Autodesk Fusion 360 part; units mm, degrees
(part 2 of 2)
  arc A402 (23.1836, 18.6599) -> (23.1836, 18.8885) centre (23.1836, 18.7742) ccw
  arc A403 (35.7225, 18.2179) -> (35.7225, 18.4465) centre (35.7225, 18.3322) ccw
  arc A404 (35.7225, 18.2179) -> (35.7225, 18.4465) centre (35.7225, 18.3322) ccw
  arc A405 (35.7225, 18.4465) -> (35.7225, 18.2179) centre (35.7225, 18.3322) ccw
  arc A406 (25.9333, 19.1335) -> (25.9333, 19.3621) centre (25.9333, 19.2478) ccw
  arc A407 (35.7225, 18.4465) -> (35.7225, 18.2179) centre (35.7225, 18.3322) ccw
  arc A408 (25.9333, 19.3621) -> (25.9333, 19.1335) centre (25.9333, 19.2478) ccw
  arc A409 (25.9333, 19.3621) -> (25.9333, 19.1335) centre (25.9333, 19.2478) ccw
  arc A410 (25.9333, 19.1335) -> (25.9333, 19.3621) centre (25.9333, 19.2478) ccw
  arc A411 (35.725, 17.5677) -> (35.725, 17.7963) centre (35.725, 17.682) ccw
  arc A412 (35.725, 17.5677) -> (35.725, 17.7963) centre (35.725, 17.682) ccw
  arc A413 (35.725, 17.7963) -> (35.725, 17.5677) centre (35.725, 17.682) ccw
  arc A414 (25.688, 16.6838) -> (25.688, 16.9124) centre (25.688, 16.7981) ccw
  arc A415 (35.725, 17.7963) -> (35.725, 17.5677) centre (35.725, 17.682) ccw
  arc A416 (25.688, 16.9124) -> (25.688, 16.6838) centre (25.688, 16.7981) ccw
  arc A417 (25.688, 16.9124) -> (25.688, 16.6838) centre (25.688, 16.7981) ccw
  arc A418 (25.688, 16.6838) -> (25.688, 16.9124) centre (25.688, 16.7981) ccw
  arc A419 (35.0722, 17.5652) -> (35.0722, 17.7938) centre (35.0722, 17.6795) ccw
  arc A420 (35.0722, 17.5652) -> (35.0722, 17.7938) centre (35.0722, 17.6795) ccw
  arc A421 (35.0722, 17.7938) -> (35.0722, 17.5652) centre (35.0722, 17.6795) ccw
  arc A422 (23.9761, 16.9835) -> (23.9761, 17.2121) centre (23.9761, 17.0978) ccw
  arc A423 (35.0722, 17.7938) -> (35.0722, 17.5652) centre (35.0722, 17.6795) ccw
  arc A424 (23.9761, 17.2121) -> (23.9761, 16.9835) centre (23.9761, 17.0978) ccw
  arc A425 (23.9761, 17.2121) -> (23.9761, 16.9835) centre (23.9761, 17.0978) ccw
  arc A426 (23.9761, 16.9835) -> (23.9761, 17.2121) centre (23.9761, 17.0978) ccw
  arc A427 (35.0697, 18.2205) -> (35.0697, 18.4491) centre (35.0697, 18.3348) ccw
  arc A428 (35.0697, 18.2205) -> (35.0697, 18.4491) centre (35.0697, 18.3348) ccw
  arc A429 (35.0697, 18.4491) -> (35.0697, 18.2205) centre (35.0697, 18.3348) ccw
  arc A430 (23.9735, 18.5964) -> (23.9735, 18.825) centre (23.9735, 18.7107) ccw
  arc A431 (35.0697, 18.4491) -> (35.0697, 18.2205) centre (35.0697, 18.3348) ccw
  arc A432 (23.9735, 18.825) -> (23.9735, 18.5964) centre (23.9735, 18.7107) ccw
  arc A433 (23.9735, 18.825) -> (23.9735, 18.5964) centre (23.9735, 18.7107) ccw
  arc A434 (23.9735, 18.5964) -> (23.9735, 18.825) centre (23.9735, 18.7107) ccw
  arc A435 (35.7197, 16.2697) -> (35.7197, 16.4983) centre (35.7197, 16.384) ccw
  arc A436 (35.7197, 16.2697) -> (35.7197, 16.4983) centre (35.7197, 16.384) ccw
  arc A437 (35.7197, 16.4983) -> (35.7197, 16.2697) centre (35.7197, 16.384) ccw
  arc A438 (28.5862, 13.2903) -> (28.5862, 13.5189) centre (28.5862, 13.4046) ccw
  arc A439 (35.7197, 16.4983) -> (35.7197, 16.2697) centre (35.7197, 16.384) ccw
  arc A440 (28.5862, 13.5189) -> (28.5862, 13.2903) centre (28.5862, 13.4046) ccw
  arc A441 (28.5862, 13.5189) -> (28.5862, 13.2903) centre (28.5862, 13.4046) ccw
  arc A442 (28.5862, 13.2903) -> (28.5862, 13.5189) centre (28.5862, 13.4046) ccw
  arc A443 (34.422, 17.5626) -> (34.422, 17.7912) centre (34.422, 17.6769) ccw
  arc A444 (34.422, 17.5626) -> (34.422, 17.7912) centre (34.422, 17.6769) ccw
  arc A445 (34.422, 17.7912) -> (34.422, 17.5626) centre (34.422, 17.6769) ccw
  arc A446 (23.9812, 17.9106) -> (23.9812, 18.1392) centre (23.9812, 18.0249) ccw
  arc A447 (34.422, 17.7912) -> (34.422, 17.5626) centre (34.422, 17.6769) ccw
  arc A448 (23.9812, 18.1392) -> (23.9812, 17.9106) centre (23.9812, 18.0249) ccw
  arc A449 (23.9812, 18.1392) -> (23.9812, 17.9106) centre (23.9812, 18.0249) ccw
  arc A450 (23.9812, 17.9106) -> (23.9812, 18.1392) centre (23.9812, 18.0249) ccw
  arc A451 (33.1215, 17.5652) -> (33.1215, 17.7938) centre (33.1215, 17.6795) ccw
  arc A452 (33.1215, 17.5652) -> (33.1215, 17.7938) centre (33.1215, 17.6795) ccw
  arc A453 (33.1215, 17.7938) -> (33.1215, 17.5652) centre (33.1215, 17.6795) ccw
  arc A454 (23.1836, 17.0597) -> (23.1836, 17.2883) centre (23.1836, 17.174) ccw
  arc A455 (33.1215, 17.7938) -> (33.1215, 17.5652) centre (33.1215, 17.6795) ccw
  arc A456 (23.1836, 17.2883) -> (23.1836, 17.0597) centre (23.1836, 17.174) ccw
  arc A457 (23.1836, 17.2883) -> (23.1836, 17.0597) centre (23.1836, 17.174) ccw
  arc A458 (23.1836, 17.0597) -> (23.1836, 17.2883) centre (23.1836, 17.174) ccw
  arc A459 (35.071, 16.2647) -> (35.071, 16.4933) centre (35.071, 16.379) ccw
  arc A460 (35.071, 16.2647) -> (35.071, 16.4933) centre (35.071, 16.379) ccw
  arc A461 (35.071, 16.4933) -> (35.071, 16.2647) centre (35.071, 16.379) ccw
  arc A462 (24.7826, 14.6455) -> (24.7826, 14.8741) centre (24.7826, 14.7598) ccw
  arc A463 (35.071, 16.4933) -> (35.071, 16.2647) centre (35.071, 16.379) ccw
  arc A464 (24.7826, 14.8741) -> (24.7826, 14.6455) centre (24.7826, 14.7598) ccw
  arc A465 (24.7826, 14.8741) -> (24.7826, 14.6455) centre (24.7826, 14.7598) ccw
  arc A466 (24.7826, 14.6455) -> (24.7826, 14.8741) centre (24.7826, 14.7598) ccw
  arc A467 (34.4207, 16.2647) -> (34.4207, 16.4933) centre (34.4207, 16.379) ccw
  arc A468 (34.4207, 16.2647) -> (34.4207, 16.4933) centre (34.4207, 16.379) ccw
  arc A469 (34.4207, 16.4933) -> (34.4207, 16.2647) centre (34.4207, 16.379) ccw
  arc A470 (25.7236, 14.954) -> (25.7236, 15.1826) centre (25.7236, 15.0683) ccw
  arc A471 (34.4207, 16.4933) -> (34.4207, 16.2647) centre (34.4207, 16.379) ccw
  arc A472 (25.7236, 15.1826) -> (25.7236, 14.954) centre (25.7236, 15.0683) ccw
  arc A473 (25.7236, 15.1826) -> (25.7236, 14.954) centre (25.7236, 15.0683) ccw
  arc A474 (25.7236, 14.954) -> (25.7236, 15.1826) centre (25.7236, 15.0683) ccw
  arc A475 (33.7705, 16.2647) -> (33.7705, 16.4933) centre (33.7705, 16.379) ccw
  arc A476 (33.7705, 16.2647) -> (33.7705, 16.4933) centre (33.7705, 16.379) ccw
  arc A477 (33.7705, 16.4933) -> (33.7705, 16.2647) centre (33.7705, 16.379) ccw
  arc A478 (25.7035, 15.8285) -> (25.7035, 16.0571) centre (25.7035, 15.9428) ccw
  arc A479 (33.7705, 16.4933) -> (33.7705, 16.2647) centre (33.7705, 16.379) ccw
  arc A480 (25.7035, 16.0571) -> (25.7035, 15.8285) centre (25.7035, 15.9428) ccw
  arc A481 (25.7035, 16.0571) -> (25.7035, 15.8285) centre (25.7035, 15.9428) ccw
  arc A482 (25.7035, 15.8285) -> (25.7035, 16.0571) centre (25.7035, 15.9428) ccw
  arc A483 (30.1007, 15.5434) -> (30.1007, 15.772) centre (30.1007, 15.6577) ccw
  arc A484 (30.1007, 15.5434) -> (30.1007, 15.772) centre (30.1007, 15.6577) ccw
  arc A485 (30.1007, 15.772) -> (30.1007, 15.5434) centre (30.1007, 15.6577) ccw
  arc A486 (33.7678, 15.6185) -> (33.7678, 15.8471) centre (33.7678, 15.7328) ccw
  arc A487 (30.1007, 15.772) -> (30.1007, 15.5434) centre (30.1007, 15.6577) ccw
  arc A488 (33.7678, 15.8471) -> (33.7678, 15.6185) centre (33.7678, 15.7328) ccw
  arc A489 (33.7678, 15.8471) -> (33.7678, 15.6185) centre (33.7678, 15.7328) ccw
  arc A490 (33.7678, 15.6185) -> (33.7678, 15.8471) centre (33.7678, 15.7328) ccw
  arc A491 (3.3894, 11.7474) -> (3.3894, 11.976) centre (3.3894, 11.8617) ccw
  arc A492 (3.3894, 11.7474) -> (3.3894, 11.976) centre (3.3894, 11.8617) ccw
  arc A493 (3.3894, 11.976) -> (3.3894, 11.7474) centre (3.3894, 11.8617) ccw
  arc A494 (3.3894, 11.976) -> (3.3894, 11.7474) centre (3.3894, 11.8617) ccw
  arc A495 (9.0206, 4.1402) -> (9.0206, 4.3688) centre (9.0206, 4.2545) ccw
  arc A496 (9.0206, 4.1402) -> (9.0206, 4.3688) centre (9.0206, 4.2545) ccw
  arc A497 (9.0206, 4.3688) -> (9.0206, 4.1402) centre (9.0206, 4.2545) ccw
  arc A498 (9.0206, 4.3688) -> (9.0206, 4.1402) centre (9.0206, 4.2545) ccw
  arc A499 (17.7429, 2.921) -> (17.7429, 3.1496) centre (17.7429, 3.0353) ccw
  arc A500 (17.7429, 2.921) -> (17.7429, 3.1496) centre (17.7429, 3.0353) ccw
  arc A501 (17.7429, 3.1496) -> (17.7429, 2.921) centre (17.7429, 3.0353) ccw
  arc A502 (17.7429, 3.1496) -> (17.7429, 2.921) centre (17.7429, 3.0353) ccw
  arc A503 (19.4676, 1.7399) -> (19.4676, 1.9685) centre (19.4676, 1.8542) ccw
  arc A504 (19.4676, 1.7399) -> (19.4676, 1.9685) centre (19.4676, 1.8542) ccw
  arc A505 (19.4676, 1.9685) -> (19.4676, 1.7399) centre (19.4676, 1.8542) ccw
  arc A506 (19.4676, 1.9685) -> (19.4676, 1.7399) centre (19.4676, 1.8542) ccw
  arc A507 (17.9778, 2.353) -> (17.9778, 2.5816) centre (17.9778, 2.4673) ccw
  arc A508 (17.9778, 2.353) -> (17.9778, 2.5816) centre (17.9778, 2.4673) ccw
  arc A509 (17.9778, 2.5816) -> (17.9778, 2.353) centre (17.9778, 2.4673) ccw
  arc A510 (17.9778, 2.5816) -> (17.9778, 2.353) centre (17.9778, 2.4673) ccw
  arc A511 (26.3452, 7.328) -> (26.3452, 7.5566) centre (26.3452, 7.4423) ccw
  arc A512 (26.3452, 7.328) -> (26.3452, 7.5566) centre (26.3452, 7.4423) ccw
  arc A513 (26.3452, 7.5566) -> (26.3452, 7.328) centre (26.3452, 7.4423) ccw
  arc A514 (26.3452, 7.5566) -> (26.3452, 7.328) centre (26.3452, 7.4423) ccw
  arc A515 (27.8558, 3.5938) -> (27.8558, 3.8224) centre (27.8558, 3.7081) ccw
  arc A516 (27.8558, 3.5938) -> (27.8558, 3.8224) centre (27.8558, 3.7081) ccw
  arc A517 (27.8558, 3.8224) -> (27.8558, 3.5938) centre (27.8558, 3.7081) ccw
  arc A518 (27.8558, 3.8224) -> (27.8558, 3.5938) centre (27.8558, 3.7081) ccw
  arc A519 (29.1578, 5.5427) -> (29.1578, 5.7713) centre (29.1578, 5.657) ccw
  arc A520 (29.1578, 5.5427) -> (29.1578, 5.7713) centre (29.1578, 5.657) ccw
  arc A521 (29.1578, 5.7713) -> (29.1578, 5.5427) centre (29.1578, 5.657) ccw
  arc A522 (29.1578, 5.7713) -> (29.1578, 5.5427) centre (29.1578, 5.657) ccw
  arc A523 (38.383, 26.0147) -> (38.383, 26.2433) centre (38.383, 26.129) ccw
  arc A524 (38.383, 26.0147) -> (38.383, 26.2433) centre (38.383, 26.129) ccw
  arc A525 (38.383, 26.2433) -> (38.383, 26.0147) centre (38.383, 26.129) ccw
  arc A526 (38.383, 26.2433) -> (38.383, 26.0147) centre (38.383, 26.129) ccw
  arc A527 (38.3794, 24.6151) -> (38.3794, 24.8437) centre (38.3794, 24.7294) ccw
  arc A528 (38.3794, 24.6151) -> (38.3794, 24.8437) centre (38.3794, 24.7294) ccw
  arc A529 (38.3794, 24.8437) -> (38.3794, 24.6151) centre (38.3794, 24.7294) ccw
  arc A530 (38.3794, 24.8437) -> (38.3794, 24.6151) centre (38.3794, 24.7294) ccw
  arc A531 (29.1551, 6.1936) -> (29.1551, 6.4222) centre (29.1551, 6.3079) ccw
  arc A532 (29.1551, 6.4222) -> (29.1551, 6.1936) centre (29.1551, 6.3079) ccw
component "Front" placed x (1, 0, 0) y (0, 1, 0) z (0, 0, 1) at (0, 0, 0)
component "Back" placed x (1, 0, 0) y (0, 1, 0) z (0, 0, 1) at (0, 0, 0)
component "Battery" placed x (1, 0, 0) y (0, 1, 0) z (0, 0, 1) at (21.9275, 16.325, 1.5)
component "Board" placed x (1, 0, 0) y (0, 1, 0) z (0, 0, 1) at (0, 0, 12.7)
component "PCB" placed x (1, 0, 0) y (0, 1, 0) z (0, 0, 1) at (0, 0, 0)
component "Component" placed x (1, 0, 0) y (0, 1, 0) z (0, 0, 1) at (0, 0, 22) in component "Front"
equation "BoardHeight = 32.65 mm"
equation "BoardWidth = 43.855 mm"
equation "EnclosureThickness = 1.5 mm"
equation "ImageSensorX = 33.5424 mm"
equation "ImageSensorY = 17.392 mm"
equation "MotionSensorX = 6.2926 mm"
equation "MotionSensorY = 17.392 mm"
equation "LensHoleDiameter = 15.1 mm + 0.2 mm + EnclosureMfgTol"
equation "MotionSensorDiameter = 10.4 mm + 0.5 mm + EnclosureMfgTol"
equation "LensExtrusionThickness = 2 mm"
equation "LensExtrusionDepth = 6 mm"
equation "OuterEdgeRadius = 6 mm"
equation "BoardRadius = 4.75 mm"
equation "MountPoint1X = 1.89 mm"
equation "MountPoint1Y = 8.172 mm"
equation "MountPointDepth = 6 mm + 0.2 mm"
equation "MountPoint2X = 34.3063 mm"
equation "MountPoint2Y = 1.90778125 mm"
equation "MountPoint3X = 41.97198125 mm"
equation "MountPoint3Y = 25.833 mm"
equation "MountPoint4X = 1.94 mm"
equation "MountPoint4Y = 28.4 mm"
equation "BackplateMountPointDepth = 5 mm"
equation "BackplateMountPointWidth = 1.5 mm"
equation "BackplateMountPointChamfer = BackplateMountPointWidth"
equation "HoleDiameter = 1.3 mm"
equation "BatteryWidth = 40 mm"
equation "BatteryHeight = 30 mm"
equation "BatteryThickness = 11 mm + 0.2 mm"
equation "BackplateOverlap = 0.2 mm"
equation "BackplateHoleOffset = 0.1 mm"
equation "ScrewHeadDiameter = 3 mm"
equation "ScrewHeadHeight = 1 mm"
equation "BackplateThickness = 1.5 mm"
equation "EnclosureDepth = EnclosureThickness + MountPointDepth + BoardThickness + BatteryThickness + BackplateThickness"
equation "BoardThickness = 3.1 mm"
equation "BoardEnclosureGap = 0.15 mm"
equation "USBCReceptacleCutoutWidth = USBCReceptacleWidth + USBCReceptacleTolerance + 2 * EnclosureMfgTol"
equation "USBCReceptacleCutoutHeight = USBCReceptacleHeight + USBCReceptacleTolerance + 2 * EnclosureMfgTol"
equation "USBCReceptacleCutoutRadius = 2.4 mm / 2 - 0.2 mm"
equation "USBCReceptacleY = 5.25348125 mm"
equation "USBCReceptacleWidth = 3.16 mm"
equation "d329 = BoardWidth"
equation "d330 = BoardHeight"
equation "d331 = BoardRadius"
equation "d332 = BoardEnclosureGap"
equation "d333 = EnclosureThickness"
equation "d334 = EnclosureDepth"
equation "d336 = BoardEnclosureGap + BackplateOverlap"
equation "d337 = BoardEnclosureGap + BackplateOverlap + 0.15 mm"
equation "d350 = MotionSensorX"
equation "d351 = MotionSensorY"
equation "d352 = ImageSensorX"
equation "d353 = ImageSensorY"
equation "d354 = EnclosureThickness"
equation "d363 = MotionSensorDiameter"
equation "d366 = LensHoleDiameter"
equation "d368 = LensHoleDiameter"
equation "d369 = LensExtrusionThickness"
equation "d370 = LensExtrusionDepth"
equation "d372 = EnclosureThickness"
equation "MountPointWidth = 3 mm"
equation "MountPointHeight = 3 mm"
equation "MountPointRadius = 1.5 mm"
equation "d404 = MountPointHeight"
equation "d407 = MountPointHeight"
equation "d409 = MountPointWidth"
equation "d411 = MountPointHeight"
equation "d412 = MountPoint1X"
equation "d413 = MountPoint1Y"
equation "d414 = MountPoint2X"
equation "d415 = MountPoint2Y"
equation "d416 = MountPoint3X"
equation "d417 = MountPoint3Y"
equation "d418 = MountPoint4X"
equation "d419 = MountPoint4Y"
equation "d420 = -MountPointDepth"
equation "d422 = MountPointRadius"
equation "d423 = MountPointDepth"
equation "d424 = HoleDiameter"
equation "d426 = BackplateThickness"
equation "d443 = BatteryWidth"
equation "d444 = BatteryHeight"
equation "d445 = BatteryThickness"
equation "d448 = BackplateMountPointWidth"
equation "d452 = BackplateHoleOffset"
equation "d453 = EnclosureThickness"
equation "d454 = BackplateMountPointDepth"
equation "d461 = ScrewHeadDiameter"
equation "d462 = ScrewHeadDiameter / 2"
equation "d463 = ScrewHeadDiameter / 3"
equation "d465 = ScrewHeadHeight - 0.3 mm"
equation "d467 = ScrewHeadHeight - 0.3 mm"
equation "d473 = EnclosureThickness + BackplateMountPointDepth + 2 mm"
equation "d474 = HoleDiameter"
equation "d476 = EnclosureThickness + BackplateMountPointDepth + 2 mm"
equation "d477 = HoleDiameter"
equation "d479 = BoardThickness"
equation "d492 = USBCReceptacleCutoutWidth"
equation "d493 = USBCReceptacleCutoutHeight"
equation "d497 = USBCReceptacleCutoutRadius"
equation "d498 = USBCReceptacleCutoutRadius"
equation "d499 = USBCReceptacleCutoutRadius"
equation "d502 = EnclosureMfgTol"
equation "d505 = -USBCReceptacleY"
equation "USBCReceptacleHeight = 8.94 mm"
equation "USBCReceptacleTolerance = 0.2 mm"
equation "EnclosureMfgTol = 0.1 mm"
equation "d509 = HoleDiameter"
equation "d510 = HoleDiameter * 2"
equation "d511 = BackplateThickness"
equation "d513 = BackplateMountPointChamfer"
named bodies: "Body", "Front", "LensExtrusion", "MountPoint4", "MountPoint1", "MountPoint3", "MountPoint2", "USBCPlugCutout"
